Autodesk Inventor part; units mm, degrees
(part 2 of 3)
  line L279 (-5.846, -1.6903) -> (-6.0548, -1.6903)
  line L280 (-6.0548, -1.6903) -> (-6.3396, -0.5285)
  line L281 (-6.3396, -0.5285) -> (-6.6164, -1.6903)
  line L282 (-6.6164, -1.6903) -> (-6.8229, -1.6903)
  line L283 (-6.8229, -1.6903) -> (-7.1802, -0.2903)
  line L284 (-7.1802, -0.2903) -> (-6.9885, -0.2903)
  line L285 (-6.9885, -0.2903) -> (-6.7071, -1.4509)
  line L286 (-6.7071, -1.4509) -> (-6.4281, -0.2903)
  line L287 (-6.4281, -0.2903) -> (-6.2386, -0.2903)
  line L288 (-6.2386, -0.2903) -> (-5.9572, -1.4645)
  line L289 (-5.9572, -1.4645) -> (-5.677, -0.2903)
  line L290 (-5.677, -0.2903) -> (-5.4943, -0.2903)
  spline S281 degree 2 poles (-4.7558, -1.5791) (-4.7773, -1.595) (-4.8499, -1.6517) (-4.884, -1.6687) knots 0 0 0 1 2 2 2
  spline S282 degree 2 poles (-4.884, -1.6687) (-4.9305, -1.6937) (-5.0178, -1.7198) (-5.0973, -1.7198) knots 0 0 0 1 2 2 2
  spline S283 degree 2 poles (-5.0973, -1.7198) (-5.1619, -1.7198) (-5.2788, -1.671) (-5.323, -1.6268) knots 0 0 0 1 2 2 2
  spline S284 degree 2 poles (-5.323, -1.6268) (-5.365, -1.5836) (-5.4161, -1.4566) (-5.4161, -1.3862) knots 0 0 0 1 2 2 2
  spline S285 degree 2 poles (-5.4161, -1.3862) (-5.4161, -1.2773) (-5.3242, -1.123) (-5.2243, -1.0788) knots 0 0 0 1 2 2 2
  spline S286 degree 2 poles (-5.2243, -1.0788) (-5.1358, -1.0379) (-4.8953, -1.0073) (-4.7558, -0.9994) knots 0 0 0 1 2 2 2
  line L291 (-4.7558, -0.9994) -> (-4.7558, -0.9653)
  spline S287 degree 2 poles (-4.7558, -0.9653) (-4.7558, -0.9041) (-4.7932, -0.8281) (-4.8272, -0.8065) knots 0 0 0 1 2 2 2
  spline S288 degree 2 poles (-4.8272, -0.8065) (-4.8613, -0.7849) (-4.9588, -0.7713) (-5.011, -0.7713) knots 0 0 0 1 2 2 2
  spline S289 degree 2 poles (-5.011, -0.7713) (-5.0723, -0.7713) (-5.2379, -0.8076) (-5.3208, -0.8428) knots 0 0 0 1 2 2 2
  line L292 (-5.3208, -0.8428) -> (-5.331, -0.8428)
  line L293 (-5.331, -0.8428) -> (-5.331, -0.6624)
  spline S290 degree 2 poles (-5.331, -0.6624) (-5.2822, -0.6488) (-5.0995, -0.6148) (-5.0099, -0.6148) knots 0 0 0 1 2 2 2
  spline S291 degree 2 poles (-5.0099, -0.6148) (-4.901, -0.6148) (-4.7524, -0.6488) (-4.6934, -0.6931) knots 0 0 0 1 2 2 2
  spline S292 degree 2 poles (-4.6934, -0.6931) (-4.6355, -0.7362) (-4.5788, -0.8734) (-4.5788, -0.9721) knots 0 0 0 1 2 2 2
  line L294 (-4.5788, -0.9721) -> (-4.5788, -1.6903)
  line L295 (-4.5788, -1.6903) -> (-4.7558, -1.6903)
  line L296 (-4.7558, -1.6903) -> (-4.7558, -1.5791)
  line L297 (-4.7558, -1.4316) -> (-4.7558, -1.1401)
  spline S293 degree 2 poles (-4.7558, -1.1401) (-4.8193, -1.1457) (-5.011, -1.165) (-5.0712, -1.1832) knots 0 0 0 1 2 2 2
  spline S294 degree 2 poles (-5.0712, -1.1832) (-5.1415, -1.2047) (-5.2334, -1.2943) (-5.2334, -1.3738) knots 0 0 0 1 2 2 2
  spline S295 degree 2 poles (-5.2334, -1.3738) (-5.2334, -1.4645) (-5.1313, -1.5564) (-5.0337, -1.5564) knots 0 0 0 1 2 2 2
  spline S296 degree 2 poles (-5.0337, -1.5564) (-4.9509, -1.5564) (-4.8148, -1.4849) (-4.7558, -1.4316) knots 0 0 0 1 2 2 2
  line L298 (-3.5055, -0.6397) -> (-3.9015, -1.6903)
  line L299 (-3.9015, -1.6903) -> (-4.0603, -1.6903)
  line L300 (-4.0603, -1.6903) -> (-4.4529, -0.6397)
  line L301 (-4.4529, -0.6397) -> (-4.2611, -0.6397)
  line L302 (-4.2611, -0.6397) -> (-3.9741, -1.4486)
  line L303 (-3.9741, -1.4486) -> (-3.6893, -0.6397)
  line L304 (-3.6893, -0.6397) -> (-3.5055, -0.6397)
  spline S297 degree 2 poles (-2.9156, -1.7141) (-3.1674, -1.7141) (-3.4443, -1.4316) (-3.4443, -1.1707) knots 0 0 0 1 2 2 2
  spline S298 degree 2 poles (-3.4443, -1.1707) (-3.4443, -0.9143) (-3.1754, -0.6102) (-2.9587, -0.6102) knots 0 0 0 1 2 2 2
  spline S299 degree 2 poles (-2.9587, -0.6102) (-2.8611, -0.6102) (-2.7102, -0.667) (-2.6546, -0.7271) knots 0 0 0 1 2 2 2
  spline S300 degree 2 poles (-2.6546, -0.7271) (-2.5979, -0.7872) (-2.5378, -0.9608) (-2.5378, -1.0867) knots 0 0 0 1 2 2 2
  line L305 (-2.5378, -1.0867) -> (-2.5378, -1.1832)
  line L306 (-2.5378, -1.1832) -> (-3.265, -1.1832)
  spline S301 degree 2 poles (-3.265, -1.1832) (-3.265, -1.3658) (-3.0812, -1.5598) (-2.9178, -1.5598) knots 0 0 0 1 2 2 2
  spline S302 degree 2 poles (-2.9178, -1.5598) (-2.86, -1.5598) (-2.7477, -1.5337) (-2.7023, -1.5133) knots 0 0 0 1 2 2 2
  spline S303 degree 2 poles (-2.7023, -1.5133) (-2.6546, -1.4906) (-2.5888, -1.4509) (-2.5673, -1.4328) knots 0 0 0 1 2 2 2
  line L307 (-2.5673, -1.4328) -> (-2.5571, -1.4328)
  line L308 (-2.5571, -1.4328) -> (-2.5571, -1.6256)
  spline S304 degree 2 poles (-2.5571, -1.6256) (-2.5877, -1.6381) (-2.6807, -1.6744) (-2.717, -1.6846) knots 0 0 0 1 2 2 2
  spline S305 degree 2 poles (-2.717, -1.6846) (-2.7681, -1.6994) (-2.852, -1.7141) (-2.9156, -1.7141) knots 0 0 0 1 2 2 2
  spline S306 degree 2 poles (-2.7102, -1.0482) (-2.7125, -0.9767) (-2.742, -0.8723) (-2.7704, -0.8371) knots 0 0 0 1 2 2 2
  spline S307 degree 2 poles (-2.7704, -0.8371) (-2.801, -0.7974) (-2.8974, -0.7554) (-2.9689, -0.7554) knots 0 0 0 1 2 2 2
  spline S308 degree 2 poles (-2.9689, -0.7554) (-3.0392, -0.7554) (-3.1379, -0.7974) (-3.1788, -0.8383) knots 0 0 0 1 2 2 2
  spline S309 degree 2 poles (-3.1788, -0.8383) (-3.2185, -0.8802) (-3.2593, -0.9812) (-3.265, -1.0482) knots 0 0 0 1 2 2 2
  line L309 (-3.265, -1.0482) -> (-2.7102, -1.0482)
  line L310 (-2.1781, -1.6903) -> (-2.3551, -1.6903)
  line L311 (-2.3551, -1.6903) -> (-2.3551, -0.2279)
  line L312 (-2.3551, -0.2279) -> (-2.1781, -0.2279)
  line L313 (-2.1781, -0.2279) -> (-2.1781, -1.6903)
  spline S310 degree 2 poles (-1.4623, -1.7141) (-1.7141, -1.7141) (-1.9909, -1.4316) (-1.9909, -1.1707) knots 0 0 0 1 2 2 2
  spline S311 degree 2 poles (-1.9909, -1.1707) (-1.9909, -0.9143) (-1.7221, -0.6102) (-1.5054, -0.6102) knots 0 0 0 1 2 2 2
  spline S312 degree 2 poles (-1.5054, -0.6102) (-1.4078, -0.6102) (-1.2569, -0.667) (-1.2013, -0.7271) knots 0 0 0 1 2 2 2
  spline S313 degree 2 poles (-1.2013, -0.7271) (-1.1446, -0.7872) (-1.0845, -0.9608) (-1.0845, -1.0867) knots 0 0 0 1 2 2 2
  line L314 (-1.0845, -1.0867) -> (-1.0845, -1.1832)
  line L315 (-1.0845, -1.1832) -> (-1.8117, -1.1832)
  spline S314 degree 2 poles (-1.8117, -1.1832) (-1.8117, -1.3658) (-1.6279, -1.5598) (-1.4645, -1.5598) knots 0 0 0 1 2 2 2
  spline S315 degree 2 poles (-1.4645, -1.5598) (-1.4067, -1.5598) (-1.2943, -1.5337) (-1.249, -1.5133) knots 0 0 0 1 2 2 2
  spline S316 degree 2 poles (-1.249, -1.5133) (-1.2013, -1.4906) (-1.1355, -1.4509) (-1.114, -1.4328) knots 0 0 0 1 2 2 2
  line L316 (-1.114, -1.4328) -> (-1.1037, -1.4328)
  line L317 (-1.1037, -1.4328) -> (-1.1037, -1.6256)
  spline S317 degree 2 poles (-1.1037, -1.6256) (-1.1344, -1.6381) (-1.2274, -1.6744) (-1.2637, -1.6846) knots 0 0 0 1 2 2 2
  spline S318 degree 2 poles (-1.2637, -1.6846) (-1.3148, -1.6994) (-1.3987, -1.7141) (-1.4623, -1.7141) knots 0 0 0 1 2 2 2
  spline S319 degree 2 poles (-1.2569, -1.0482) (-1.2592, -0.9767) (-1.2887, -0.8723) (-1.317, -0.8371) knots 0 0 0 1 2 2 2
  spline S320 degree 2 poles (-1.317, -0.8371) (-1.3477, -0.7974) (-1.4441, -0.7554) (-1.5156, -0.7554) knots 0 0 0 1 2 2 2
  spline S321 degree 2 poles (-1.5156, -0.7554) (-1.5859, -0.7554) (-1.6846, -0.7974) (-1.7255, -0.8383) knots 0 0 0 1 2 2 2
  spline S322 degree 2 poles (-1.7255, -0.8383) (-1.7652, -0.8802) (-1.806, -0.9812) (-1.8117, -1.0482) knots 0 0 0 1 2 2 2
  line L318 (-1.8117, -1.0482) -> (-1.2569, -1.0482)
  line L319 (-0.0804, -1.6903) -> (-0.2574, -1.6903)
  line L320 (-0.2574, -1.6903) -> (-0.2574, -1.0913)
  spline S323 degree 2 poles (-0.2574, -1.0913) (-0.2574, -1.0187) (-0.271, -0.8939) (-0.2914, -0.8564) knots 0 0 0 1 2 2 2
  spline S324 degree 2 poles (-0.2914, -0.8564) (-0.313, -0.8167) (-0.3901, -0.7781) (-0.4559, -0.7781) knots 0 0 0 1 2 2 2
  spline S325 degree 2 poles (-0.4559, -0.7781) (-0.5217, -0.7781) (-0.6613, -0.8485) (-0.7282, -0.9052) knots 0 0 0 1 2 2 2
  line L321 (-0.7282, -0.9052) -> (-0.7282, -1.6903)
  line L322 (-0.7282, -1.6903) -> (-0.9052, -1.6903)
  line L323 (-0.9052, -1.6903) -> (-0.9052, -0.6397)
  line L324 (-0.9052, -0.6397) -> (-0.7282, -0.6397)
  line L325 (-0.7282, -0.6397) -> (-0.7282, -0.7566)
  spline S326 degree 2 poles (-0.7282, -0.7566) (-0.6488, -0.6851) (-0.4956, -0.6102) (-0.4094, -0.6102) knots 0 0 0 1 2 2 2
  spline S327 degree 2 poles (-0.4094, -0.6102) (-0.2551, -0.6102) (-0.0804, -0.8144) (-0.0804, -1.0084) knots 0 0 0 1 2 2 2
  line L326 (-0.0804, -1.0084) -> (-0.0804, -1.6903)
  spline S328 degree 2 poles (0.2055, -1.8582) (0.2236, -1.8661) (0.2929, -1.8911) (0.3371, -1.9013) knots 0 0 0 1 2 2 2
  spline S329 degree 2 poles (0.3371, -1.9013) (0.3859, -1.9138) (0.4687, -1.9285) (0.5175, -1.9285) knots 0 0 0 1 2 2 2
  spline S330 degree 2 poles (0.5175, -1.9285) (0.5992, -1.9285) (0.7126, -1.8854) (0.7444, -1.8469) knots 0 0 0 1 2 2 2
  spline S331 degree 2 poles (0.7444, -1.8469) (0.775, -1.8083) (0.7989, -1.7073) (0.7989, -1.6426) knots 0 0 0 1 2 2 2
  line L327 (0.7989, -1.6426) -> (0.7989, -1.5507)
  spline S332 degree 2 poles (0.7989, -1.5507) (0.7274, -1.6131) (0.5901, -1.6721) (0.4869, -1.6721) knots 0 0 0 1 2 2 2
  spline S333 degree 2 poles (0.4869, -1.6721) (0.3076, -1.6721) (0.0954, -1.4055) (0.0954, -1.1548) knots 0 0 0 1 2 2 2
  spline S334 degree 2 poles (0.0954, -1.1548) (0.0954, -1.0243) (0.1692, -0.8224) (0.2305, -0.7509) knots 0 0 0 1 2 2 2
  spline S335 degree 2 poles (0.2305, -0.7509) (0.2895, -0.684) (0.4517, -0.6102) (0.5379, -0.6102) knots 0 0 0 1 2 2 2
  spline S336 degree 2 poles (0.5379, -0.6102) (0.6196, -0.6102) (0.7387, -0.6488) (0.7989, -0.684) knots 0 0 0 1 2 2 2
  line L328 (0.7989, -0.684) -> (0.8091, -0.6397)
  line L329 (0.8091, -0.6397) -> (0.9758, -0.6397)
  line L330 (0.9758, -0.6397) -> (0.9758, -1.57)
  spline S337 degree 2 poles (0.9758, -1.57) (0.9758, -1.8378) (0.7433, -2.0874) (0.5039, -2.0874) knots 0 0 0 1 2 2 2
  spline S338 degree 2 poles (0.5039, -2.0874) (0.4267, -2.0874) (0.2656, -2.0624) (0.1964, -2.042) knots 0 0 0 1 2 2 2
  line L331 (0.1964, -2.042) -> (0.1964, -1.8582)
  line L332 (0.1964, -1.8582) -> (0.2055, -1.8582)
  line L333 (0.7989, -1.4055) -> (0.7989, -0.8281)
  spline S339 degree 2 poles (0.7989, -0.8281) (0.733, -0.7963) (0.6219, -0.7691) (0.5663, -0.7691) knots 0 0 0 1 2 2 2
  spline S340 degree 2 poles (0.5663, -0.7691) (0.4324, -0.7691) (0.2781, -0.9665) (0.2781, -1.1514) knots 0 0 0 1 2 2 2
  spline S341 degree 2 poles (0.2781, -1.1514) (0.2781, -1.3261) (0.395, -1.5088) (0.5266, -1.5088) knots 0 0 0 1 2 2 2
  spline S342 degree 2 poles (0.5266, -1.5088) (0.5958, -1.5088) (0.741, -1.4543) (0.7989, -1.4055) knots 0 0 0 1 2 2 2
  spline S343 degree 2 poles (1.5499, -1.7107) (1.4058, -1.7107) (1.2436, -1.5462) (1.2436, -1.3681) knots 0 0 0 1 2 2 2
  line L334 (1.2436, -1.3681) -> (1.2436, -0.7861)
  line L335 (1.2436, -0.7861) -> (1.1245, -0.7861)
  line L336 (1.1245, -0.7861) -> (1.1245, -0.6397)
  line L337 (1.1245, -0.6397) -> (1.2436, -0.6397)
  line L338 (1.2436, -0.6397) -> (1.2436, -0.3379)
  line L339 (1.2436, -0.3379) -> (1.4206, -0.3379)
  line L340 (1.4206, -0.3379) -> (1.4206, -0.6397)
  line L341 (1.4206, -0.6397) -> (1.7462, -0.6397)
  line L342 (1.7462, -0.6397) -> (1.7462, -0.7861)
  line L343 (1.7462, -0.7861) -> (1.4206, -0.7861)
  line L344 (1.4206, -0.7861) -> (1.4206, -1.2864)
  spline S344 degree 2 poles (1.4206, -1.2864) (1.4206, -1.3658) (1.4262, -1.4532) (1.4455, -1.4906) knots 0 0 0 1 2 2 2
  spline S345 degree 2 poles (1.4455, -1.4906) (1.4614, -1.5235) (1.5329, -1.5564) (1.5942, -1.5564) knots 0 0 0 1 2 2 2
  spline S346 degree 2 poles (1.5942, -1.5564) (1.6373, -1.5564) (1.7178, -1.5303) (1.736, -1.5224) knots 0 0 0 1 2 2 2
  line L345 (1.736, -1.5224) -> (1.7462, -1.5224)
  line L346 (1.7462, -1.5224) -> (1.7462, -1.6812)
  spline S347 degree 2 poles (1.7462, -1.6812) (1.6963, -1.6948) (1.5942, -1.7107) (1.5499, -1.7107) knots 0 0 0 1 2 2 2
  line L347 (2.7014, -1.6903) -> (2.5245, -1.6903)
  line L348 (2.5245, -1.6903) -> (2.5245, -1.0913)
  spline S348 degree 2 poles (2.5245, -1.0913) (2.5245, -1.0187) (2.5108, -0.8939) (2.4904, -0.8564) knots 0 0 0 1 2 2 2
  spline S349 degree 2 poles (2.4904, -0.8564) (2.4689, -0.8167) (2.3917, -0.7781) (2.3259, -0.7781) knots 0 0 0 1 2 2 2
  spline S350 degree 2 poles (2.3259, -0.7781) (2.2601, -0.7781) (2.1206, -0.8485) (2.0536, -0.9052) knots 0 0 0 1 2 2 2
  line L349 (2.0536, -0.9052) -> (2.0536, -1.6903)
  line L350 (2.0536, -1.6903) -> (1.8766, -1.6903)
  line L351 (1.8766, -1.6903) -> (1.8766, -0.2279)
  line L352 (1.8766, -0.2279) -> (2.0536, -0.2279)
  line L353 (2.0536, -0.2279) -> (2.0536, -0.7566)
  spline S351 degree 2 poles (2.0536, -0.7566) (2.133, -0.6851) (2.2862, -0.6102) (2.3724, -0.6102) knots 0 0 0 1 2 2 2
  spline S352 degree 2 poles (2.3724, -0.6102) (2.5267, -0.6102) (2.7014, -0.8144) (2.7014, -1.0084) knots 0 0 0 1 2 2 2
  line L354 (2.7014, -1.0084) -> (2.7014, -1.6903)
  line L355 (3.8757, -1.6903) -> (3.651, -1.6903)
  line L356 (3.651, -1.6903) -> (3.651, -1.4225)
  line L357 (3.651, -1.4225) -> (3.8757, -1.4225)
  line L358 (3.8757, -1.4225) -> (3.8757, -1.6903)
  line L359 (3.8757, -0.9075) -> (3.651, -0.9075)
  line L360 (3.651, -0.9075) -> (3.651, -0.6397)
  line L361 (3.651, -0.6397) -> (3.8757, -0.6397)
  line L362 (3.8757, -0.6397) -> (3.8757, -0.9075)
  spline S353 degree 2 poles (5.692, -1.2365) (5.692, -1.3443) (5.6206, -1.5269) (5.5604, -1.5882) knots 0 0 0 1 2 2 2
  spline S354 degree 2 poles (5.5604, -1.5882) (5.498, -1.6529) (5.3415, -1.7198) (5.2473, -1.7198) knots 0 0 0 1 2 2 2
  spline S355 degree 2 poles (5.2473, -1.7198) (5.1531, -1.7198) (4.9977, -1.6563) (4.9387, -1.5927) knots 0 0 0 1 2 2 2
  spline S356 degree 2 poles (4.9387, -1.5927) (4.8661, -1.5167) (4.7844, -1.2614) (4.7844, -1.0754) knots 0 0 0 1 2 2 2
  spline S357 degree 2 poles (4.7844, -1.0754) (4.7844, -0.8927) (4.8593, -0.5989) (4.9376, -0.49) knots 0 0 0 1 2 2 2
  spline S358 degree 2 poles (4.9376, -0.49) (5.0136, -0.3833) (5.2541, -0.2642) (5.4118, -0.2642) knots 0 0 0 1 2 2 2
  spline S359 degree 2 poles (5.4118, -0.2642) (5.4583, -0.2642) (5.54, -0.2733) (5.5707, -0.2835) knots 0 0 0 1 2 2 2
  line L363 (5.5707, -0.2835) -> (5.5707, -0.4639)
  line L364 (5.5707, -0.4639) -> (5.5627, -0.4639)
  spline S360 degree 2 poles (5.5627, -0.4639) (5.5366, -0.4503) (5.4413, -0.4264) (5.3869, -0.4264) knots 0 0 0 1 2 2 2
  spline S361 degree 2 poles (5.3869, -0.4264) (5.2121, -0.4264) (4.9977, -0.6624) (4.9773, -0.8939) knots 0 0 0 1 2 2 2
  spline S362 degree 2 poles (4.9773, -0.8939) (5.0442, -0.8473) (5.1849, -0.7963) (5.2689, -0.7963) knots 0 0 0 1 2 2 2
  spline S363 degree 2 poles (5.2689, -0.7963) (5.3506, -0.7963) (5.4731, -0.8292) (5.54, -0.8791) knots 0 0 0 1 2 2 2
  spline S364 degree 2 poles (5.54, -0.8791) (5.6172, -0.937) (5.692, -1.1162) (5.692, -1.2365) knots 0 0 0 1 2 2 2
  spline S365 degree 2 poles (5.5014, -1.2444) (5.5014, -1.1582) (5.4561, -1.0413) (5.4061, -1.0005) knots 0 0 0 1 2 2 2
  spline S366 degree 2 poles (5.4061, -1.0005) (5.3687, -0.971) (5.2757, -0.9517) (5.2269, -0.9517) knots 0 0 0 1 2 2 2
  spline S367 degree 2 poles (5.2269, -0.9517) (5.1611, -0.9517) (5.0374, -0.9914) (4.9773, -1.0289) knots 0 0 0 1 2 2 2
  spline S368 degree 2 poles (4.9773, -1.0289) (4.9762, -1.0493) (4.9739, -1.0879) (4.9739, -1.1174) knots 0 0 0 1 2 2 2
  spline S369 degree 2 poles (4.9739, -1.1174) (4.9739, -1.2626) (5.0306, -1.4407) (5.0737, -1.4872) knots 0 0 0 1 2 2 2
  spline S370 degree 2 poles (5.0737, -1.4872) (5.1134, -1.5315) (5.1997, -1.5666) (5.2484, -1.5666) knots 0 0 0 1 2 2 2
  spline S371 degree 2 poles (5.2484, -1.5666) (5.3619, -1.5666) (5.5014, -1.4055) (5.5014, -1.2444) knots 0 0 0 1 2 2 2
  spline S372 degree 2 poles (6.2355, -0.423) (6.1844, -0.423) (6.0835, -0.448) (6.0347, -0.4673) knots 0 0 0 1 2 2 2
  spline S373 degree 2 poles (6.0347, -0.4673) (5.9893, -0.4866) (5.9224, -0.5274) (5.8963, -0.5456) knots 0 0 0 1 2 2 2
  line L365 (5.8963, -0.5456) -> (5.8849, -0.5456)
  line L366 (5.8849, -0.5456) -> (5.8849, -0.347)
  spline S374 degree 2 poles (5.8849, -0.347) (5.9462, -0.3141) (6.1561, -0.2608) (6.2502, -0.2608) knots 0 0 0 1 2 2 2
  spline S375 degree 2 poles (6.2502, -0.2608) (6.3455, -0.2608) (6.4873, -0.2994) (6.5452, -0.3402) knots 0 0 0 1 2 2 2
  spline S376 degree 2 poles (6.5452, -0.3402) (6.6065, -0.3845) (6.67, -0.5127) (6.67, -0.5989) knots 0 0 0 1 2 2 2
  spline S377 degree 2 poles (6.67, -0.5989) (6.67, -0.7146) (6.518, -0.8893) (6.4113, -0.912) knots 0 0 0 1 2 2 2
  line L367 (6.4113, -0.912) -> (6.4113, -0.9256)
  spline S378 degree 2 poles (6.4113, -0.9256) (6.4556, -0.9347) (6.5565, -0.9755) (6.5997, -1.0164) knots 0 0 0 1 2 2 2
  spline S379 degree 2 poles (6.5997, -1.0164) (6.6428, -1.0561) (6.6972, -1.1832) (6.6972, -1.2751) knots 0 0 0 1 2 2 2
  spline S380 degree 2 poles (6.6972, -1.2751) (6.6972, -1.3692) (6.6326, -1.5292) (6.5736, -1.5905) knots 0 0 0 1 2 2 2
  spline S381 degree 2 poles (6.5736, -1.5905) (6.5123, -1.654) (6.3387, -1.7198) (6.2287, -1.7198) knots 0 0 0 1 2 2 2
  spline S382 degree 2 poles (6.2287, -1.7198) (6.1232, -1.7198) (5.9167, -1.6687) (5.8463, -1.6336) knots 0 0 0 1 2 2 2
  line L368 (5.8463, -1.6336) -> (5.8463, -1.435)
  line L369 (5.8463, -1.435) -> (5.86, -1.435)
  spline S383 degree 2 poles (5.86, -1.435) (5.9189, -1.4781) (6.1186, -1.5576) (6.2173, -1.5576) knots 0 0 0 1 2 2 2
  spline S384 degree 2 poles (6.2173, -1.5576) (6.2752, -1.5576) (6.3909, -1.5213) (6.4295, -1.4793) knots 0 0 0 1 2 2 2
  spline S385 degree 2 poles (6.4295, -1.4793) (6.4669, -1.4373) (6.5066, -1.3375) (6.5066, -1.2614) knots 0 0 0 1 2 2 2
  spline S386 degree 2 poles (6.5066, -1.2614) (6.5066, -1.1854) (6.4624, -1.0867) (6.4227, -1.0584) knots 0 0 0 1 2 2 2
  spline S387 degree 2 poles (6.4227, -1.0584) (6.383, -1.03) (6.2752, -1.0084) (6.2117, -1.0084) knots 0 0 0 1 2 2 2
  line L370 (6.2117, -1.0084) -> (6.1322, -1.0084)
  line L371 (6.1322, -1.0084) -> (6.1322, -0.853)
  line L372 (6.1322, -0.853) -> (6.1946, -0.853)
  spline S388 degree 2 poles (6.1946, -0.853) (6.3206, -0.853) (6.4794, -0.7328) (6.4794, -0.6182) knots 0 0 0 1 2 2 2
  spline S389 degree 2 poles (6.4794, -0.6182) (6.4794, -0.5648) (6.4386, -0.4888) (6.4057, -0.4661) knots 0 0 0 1 2 2 2
  spline S390 degree 2 poles (6.4057, -0.4661) (6.3705, -0.4423) (6.2843, -0.423) (6.2355, -0.423) knots 0 0 0 1 2 2 2
  spline S391 degree 2 poles (7.7932, -1.2365) (7.7932, -1.3443) (7.7217, -1.5269) (7.6616, -1.5882) knots 0 0 0 1 2 2 2
  spline S392 degree 2 poles (7.6616, -1.5882) (7.5992, -1.6529) (7.4426, -1.7198) (7.3484, -1.7198) knots 0 0 0 1 2 2 2
  spline S393 degree 2 poles (7.3484, -1.7198) (7.2543, -1.7198) (7.0989, -1.6563) (7.0399, -1.5927) knots 0 0 0 1 2 2 2
  spline S394 degree 2 poles (7.0399, -1.5927) (6.9672, -1.5167) (6.8856, -1.2614) (6.8856, -1.0754) knots 0 0 0 1 2 2 2
  spline S395 degree 2 poles (6.8856, -1.0754) (6.8856, -0.8927) (6.9604, -0.5989) (7.0387, -0.49) knots 0 0 0 1 2 2 2
  spline S396 degree 2 poles (7.0387, -0.49) (7.1147, -0.3833) (7.3553, -0.2642) (7.513, -0.2642) knots 0 0 0 1 2 2 2
  spline S397 degree 2 poles (7.513, -0.2642) (7.5595, -0.2642) (7.6412, -0.2733) (7.6718, -0.2835) knots 0 0 0 1 2 2 2
  line L373 (7.6718, -0.2835) -> (7.6718, -0.4639)
  line L374 (7.6718, -0.4639) -> (7.6638, -0.4639)
  spline S398 degree 2 poles (7.6638, -0.4639) (7.6377, -0.4503) (7.5424, -0.4264) (7.488, -0.4264) knots 0 0 0 1 2 2 2
  spline S399 degree 2 poles (7.488, -0.4264) (7.3133, -0.4264) (7.0989, -0.6624) (7.0784, -0.8939) knots 0 0 0 1 2 2 2
  spline S400 degree 2 poles (7.0784, -0.8939) (7.1454, -0.8473) (7.286, -0.7963) (7.37, -0.7963) knots 0 0 0 1 2 2 2
  spline S401 degree 2 poles (7.37, -0.7963) (7.4517, -0.7963) (7.5742, -0.8292) (7.6412, -0.8791) knots 0 0 0 1 2 2 2
  spline S402 degree 2 poles (7.6412, -0.8791) (7.7183, -0.937) (7.7932, -1.1162) (7.7932, -1.2365) knots 0 0 0 1 2 2 2
  spline S403 degree 2 poles (7.6026, -1.2444) (7.6026, -1.1582) (7.5572, -1.0413) (7.5073, -1.0005) knots 0 0 0 1 2 2 2
  spline S404 degree 2 poles (7.5073, -1.0005) (7.4698, -0.971) (7.3768, -0.9517) (7.328, -0.9517) knots 0 0 0 1 2 2 2
  spline S405 degree 2 poles (7.328, -0.9517) (7.2622, -0.9517) (7.1386, -0.9914) (7.0784, -1.0289) knots 0 0 0 1 2 2 2
  spline S406 degree 2 poles (7.0784, -1.0289) (7.0773, -1.0493) (7.075, -1.0879) (7.075, -1.1174) knots 0 0 0 1 2 2 2
  spline S407 degree 2 poles (7.075, -1.1174) (7.075, -1.2626) (7.1318, -1.4407) (7.1749, -1.4872) knots 0 0 0 1 2 2 2
  spline S408 degree 2 poles (7.1749, -1.4872) (7.2146, -1.5315) (7.3008, -1.5666) (7.3496, -1.5666) knots 0 0 0 1 2 2 2
  spline S409 degree 2 poles (7.3496, -1.5666) (7.463, -1.5666) (7.6026, -1.4055) (7.6026, -1.2444) knots 0 0 0 1 2 2 2
  line L375 (8.2595, -1.6903) -> (8.0348, -1.6903)
  line L376 (8.0348, -1.6903) -> (8.0348, -1.4225)
  line L377 (8.0348, -1.4225) -> (8.2595, -1.4225)
  line L378 (8.2595, -1.4225) -> (8.2595, -1.6903)
  spline S410 degree 2 poles (8.5034, -0.7452) (8.5034, -0.6375) (8.5737, -0.4582) (8.635, -0.3935) knots 0 0 0 1 2 2 2
  spline S411 degree 2 poles (8.635, -0.3935) (8.6929, -0.3311) (8.8619, -0.2619) (8.9481, -0.2619) knots 0 0 0 1 2 2 2
  spline S412 degree 2 poles (8.9481, -0.2619) (9.0446, -0.2619) (9.2011, -0.3266) (9.259, -0.3879) knots 0 0 0 1 2 2 2
  spline S413 degree 2 poles (9.259, -0.3879) (9.3316, -0.465) (9.411, -0.7146) (9.411, -0.9063) knots 0 0 0 1 2 2 2
  spline S414 degree 2 poles (9.411, -0.9063) (9.411, -1.0799) (9.3327, -1.3908) (9.2567, -1.494) knots 0 0 0 1 2 2 2
  spline S415 degree 2 poles (9.2567, -1.494) (9.1762, -1.6029) (8.9493, -1.7175) (8.7836, -1.7175) knots 0 0 0 1 2 2 2
  spline S416 degree 2 poles (8.7836, -1.7175) (8.7462, -1.7175) (8.6611, -1.7096) (8.6248, -1.6982) knots 0 0 0 1 2 2 2
  line L379 (8.6248, -1.6982) -> (8.6248, -1.5178)
  line L380 (8.6248, -1.5178) -> (8.6339, -1.5178)
  spline S417 degree 2 poles (8.6339, -1.5178) (8.6577, -1.5315) (8.7575, -1.5553) (8.8086, -1.5553) knots 0 0 0 1 2 2 2
  spline S418 degree 2 poles (8.8086, -1.5553) (8.9924, -1.5553) (9.2023, -1.3125) (9.217, -1.0879) knots 0 0 0 1 2 2 2
  spline S419 degree 2 poles (9.217, -1.0879) (9.1421, -1.1389) (9.006, -1.1854) (8.9254, -1.1854) knots 0 0 0 1 2 2 2
  spline S420 degree 2 poles (8.9254, -1.1854) (8.8483, -1.1854) (8.7201, -1.1514) (8.6554, -1.1026) knots 0 0 0 1 2 2 2
  spline S421 degree 2 poles (8.6554, -1.1026) (8.5805, -1.0448) (8.5034, -0.8689) (8.5034, -0.7452) knots 0 0 0 1 2 2 2
  spline S422 degree 2 poles (9.2215, -0.8644) (9.2215, -0.7225) (9.1694, -0.5433) (9.1228, -0.4945) knots 0 0 0 1 2 2 2
  spline S423 degree 2 poles (9.1228, -0.4945) (9.082, -0.4491) (8.9969, -0.4151) (8.947, -0.4151) knots 0 0 0 1 2 2 2
  spline S424 degree 2 poles (8.947, -0.4151) (8.8313, -0.4151) (8.694, -0.5807) (8.694, -0.7373) knots 0 0 0 1 2 2 2
  spline S425 degree 2 poles (8.694, -0.7373) (8.694, -0.8258) (8.7394, -0.9404) (8.7893, -0.9812) knots 0 0 0 1 2 2 2
  spline S426 degree 2 poles (8.7893, -0.9812) (8.8256, -1.0107) (8.9152, -1.03) (8.9674, -1.03) knots 0 0 0 1 2 2 2
  spline S427 degree 2 poles (8.9674, -1.03) (9.0275, -1.03) (9.166, -0.988) (9.2181, -0.9529) knots 0 0 0 1 2 2 2
  spline S428 degree 2 poles (9.2181, -0.9529) (9.2193, -0.9392) (9.2215, -0.8927) (9.2215, -0.8644) knots 0 0 0 1 2 2 2
  line L381 (11.0447, -1.6903) -> (10.8677, -1.6903)
  line L382 (10.8677, -1.6903) -> (10.8677, -1.0913)
  spline S429 degree 2 poles (10.8677, -1.0913) (10.8677, -1.0187) (10.8541, -0.8939) (10.8337, -0.8564) knots 0 0 0 1 2 2 2
  spline S430 degree 2 poles (10.8337, -0.8564) (10.8121, -0.8167) (10.735, -0.7781) (10.6692, -0.7781) knots 0 0 0 1 2 2 2
  spline S431 degree 2 poles (10.6692, -0.7781) (10.6034, -0.7781) (10.4638, -0.8485) (10.3969, -0.9052) knots 0 0 0 1 2 2 2
  line L383 (10.3969, -0.9052) -> (10.3969, -1.6903)
  line L384 (10.3969, -1.6903) -> (10.2199, -1.6903)
  line L385 (10.2199, -1.6903) -> (10.2199, -0.6397)
  line L386 (10.2199, -0.6397) -> (10.3969, -0.6397)
  line L387 (10.3969, -0.6397) -> (10.3969, -0.7566)
  spline S432 degree 2 poles (10.3969, -0.7566) (10.4763, -0.6851) (10.6295, -0.6102) (10.7157, -0.6102) knots 0 0 0 1 2 2 2
  spline S433 degree 2 poles (10.7157, -0.6102) (10.87, -0.6102) (11.0447, -0.8144) (11.0447, -1.0084) knots 0 0 0 1 2 2 2
  line L388 (11.0447, -1.0084) -> (11.0447, -1.6903)
  line L389 (12.4844, -1.6903) -> (12.4844, -1.0822)
  spline S434 degree 2 poles (12.4844, -1.0822) (12.4844, -1.0096) (12.4731, -0.8859) (12.4549, -0.8519) knots 0 0 0 1 2 2 2
  spline S435 degree 2 poles (12.4549, -0.8519) (12.4368, -0.8144) (12.3676, -0.7781) (12.3074, -0.7781) knots 0 0 0 1 2 2 2
  spline S436 degree 2 poles (12.3074, -0.7781) (12.253, -0.7781) (12.1282, -0.8451) (12.0624, -0.9086) knots 0 0 0 1 2 2 2
  spline S437 degree 2 poles (12.0624, -0.9086) (12.0635, -0.9245) (12.0658, -0.9687) (12.0658, -0.9982) knots 0 0 0 1 2 2 2
  line L390 (12.0658, -0.9982) -> (12.0658, -1.6903)
  line L391 (12.0658, -1.6903) -> (11.8888, -1.6903)
  line L392 (11.8888, -1.6903) -> (11.8888, -1.0822)
  spline S438 degree 2 poles (11.8888, -1.0822) (11.8888, -1.0096) (11.8775, -0.8859) (11.8593, -0.8519) knots 0 0 0 1 2 2 2
  spline S439 degree 2 poles (11.8593, -0.8519) (11.8412, -0.8144) (11.7719, -0.7781) (11.7118, -0.7781) knots 0 0 0 1 2 2 2
  spline S440 degree 2 poles (11.7118, -0.7781) (11.6551, -0.7781) (11.5292, -0.8496) (11.4702, -0.9052) knots 0 0 0 1 2 2 2
  line L393 (11.4702, -0.9052) -> (11.4702, -1.6903)
  line L394 (11.4702, -1.6903) -> (11.2932, -1.6903)
  line L395 (11.2932, -1.6903) -> (11.2932, -0.6397)
  line L396 (11.2932, -0.6397) -> (11.4702, -0.6397)
  line L397 (11.4702, -0.6397) -> (11.4702, -0.7554)
  spline S441 degree 2 poles (11.4702, -0.7554) (11.5394, -0.6862) (11.6755, -0.6102) (11.7572, -0.6102) knots 0 0 0 1 2 2 2
  spline S442 degree 2 poles (11.7572, -0.6102) (11.8502, -0.6102) (11.9943, -0.6953) (12.0318, -0.7918) knots 0 0 0 1 2 2 2
  spline S443 degree 2 poles (12.0318, -0.7918) (12.1123, -0.7021) (12.2643, -0.6102) (12.3528, -0.6102) knots 0 0 0 1 2 2 2
  spline S444 degree 2 poles (12.3528, -0.6102) (12.4209, -0.6102) (12.5321, -0.6522) (12.5729, -0.6999) knots 0 0 0 1 2 2 2
  spline S445 degree 2 poles (12.5729, -0.6999) (12.6149, -0.7475) (12.6614, -0.8905) (12.6614, -0.9982) knots 0 0 0 1 2 2 2
  line L398 (12.6614, -0.9982) -> (12.6614, -1.6903)
  line L399 (12.6614, -1.6903) -> (12.4844, -1.6903)
  line L400 (-12.4217, -2.761) -> (-13.0729, -2.761)
  line L401 (-13.0729, -2.761) -> (-13.0729, -3.1558)
  line L402 (-13.0729, -3.1558) -> (-12.449, -3.1558)
  line L403 (-12.449, -3.1558) -> (-12.449, -3.3215)
  line L404 (-12.449, -3.3215) -> (-13.0729, -3.3215)
  line L405 (-13.0729, -3.3215) -> (-13.0729, -3.9954)
  line L406 (-13.0729, -3.9954) -> (-13.259, -3.9954)
  line L407 (-13.259, -3.9954) -> (-13.259, -2.5954)
  line L408 (-13.259, -2.5954) -> (-12.4217, -2.5954)
  line L409 (-12.4217, -2.5954) -> (-12.4217, -2.761)
  line L410 (-12.0882, -3.9954) -> (-12.2652, -3.9954)
  line L411 (-12.2652, -3.9954) -> (-12.2652, -2.9448)
  line L412 (-12.2652, -2.9448) -> (-12.0882, -2.9448)
  line L413 (-12.0882, -2.9448) -> (-12.0882, -3.9954)
  line L414 (-12.0757, -2.7701) -> (-12.2765, -2.7701)
  line L415 (-12.2765, -2.7701) -> (-12.2765, -2.5863)
  line L416 (-12.2765, -2.5863) -> (-12.0757, -2.5863)
  line L417 (-12.0757, -2.5863) -> (-12.0757, -2.7701)
  spline S446 degree 2 poles (-10.948, -3.4531) (-10.948, -3.7106) (-11.1976, -4.0249) (-11.3859, -4.0249) knots 0 0 0 1 2 2 2
  spline S447 degree 2 poles (-11.3859, -4.0249) (-11.471, -4.0249) (-11.5924, -3.9829) (-11.6514, -3.9466) knots 0 0 0 1 2 2 2
  line L418 (-11.6514, -3.9466) -> (-11.6627, -3.9954)
  line L419 (-11.6627, -3.9954) -> (-11.8284, -3.9954)
  line L420 (-11.8284, -3.9954) -> (-11.8284, -2.533)
  line L421 (-11.8284, -2.533) -> (-11.6514, -2.533)
  line L422 (-11.6514, -2.533) -> (-11.6514, -3.0548)
  spline S448 degree 2 poles (-11.6514, -3.0548) (-11.5845, -2.9947) (-11.429, -2.9153) (-11.3303, -2.9153) knots 0 0 0 1 2 2 2
  spline S449 degree 2 poles (-11.3303, -2.9153) (-11.1522, -2.9153) (-10.948, -3.2001) (-10.948, -3.4531) knots 0 0 0 1 2 2 2
  spline S450 degree 2 poles (-11.1306, -3.4667) (-11.1306, -3.2783) (-11.2452, -3.0832) (-11.3723, -3.0832) knots 0 0 0 1 2 2 2
  spline S451 degree 2 poles (-11.3723, -3.0832) (-11.4438, -3.0832) (-11.5913, -3.1513) (-11.6514, -3.2035) knots 0 0 0 1 2 2 2
  line L423 (-11.6514, -3.2035) -> (-11.6514, -3.8059)
  spline S452 degree 2 poles (-11.6514, -3.8059) (-11.5845, -3.8388) (-11.4812, -3.866) (-11.4199, -3.866) knots 0 0 0 1 2 2 2
  spline S453 degree 2 poles (-11.4199, -3.866) (-11.2849, -3.866) (-11.1306, -3.6743) (-11.1306, -3.4667) knots 0 0 0 1 2 2 2
  spline S454 degree 2 poles (-10.3081, -4.0192) (-10.56, -4.0192) (-10.8368, -3.7367) (-10.8368, -3.4757) knots 0 0 0 1 2 2 2
  spline S455 degree 2 poles (-10.8368, -3.4757) (-10.8368, -3.2193) (-10.5679, -2.9153) (-10.3512, -2.9153) knots 0 0 0 1 2 2 2
  spline S456 degree 2 poles (-10.3512, -2.9153) (-10.2537, -2.9153) (-10.1028, -2.972) (-10.0472, -3.0321) knots 0 0 0 1 2 2 2
  spline S457 degree 2 poles (-10.0472, -3.0321) (-9.9905, -3.0923) (-9.9303, -3.2659) (-9.9303, -3.3918) knots 0 0 0 1 2 2 2
  line L424 (-9.9303, -3.3918) -> (-9.9303, -3.4882)
  line L425 (-9.9303, -3.4882) -> (-10.6576, -3.4882)
  spline S458 degree 2 poles (-10.6576, -3.4882) (-10.6576, -3.6709) (-10.4738, -3.8649) (-10.3104, -3.8649) knots 0 0 0 1 2 2 2
  spline S459 degree 2 poles (-10.3104, -3.8649) (-10.2525, -3.8649) (-10.1402, -3.8388) (-10.0948, -3.8184) knots 0 0 0 1 2 2 2
  spline S460 degree 2 poles (-10.0948, -3.8184) (-10.0472, -3.7957) (-9.9814, -3.756) (-9.9598, -3.7378) knots 0 0 0 1 2 2 2
  line L426 (-9.9598, -3.7378) -> (-9.9496, -3.7378)
  line L427 (-9.9496, -3.7378) -> (-9.9496, -3.9307)
  spline S461 degree 2 poles (-9.9496, -3.9307) (-9.9802, -3.9432) (-10.0733, -3.9795) (-10.1096, -3.9897) knots 0 0 0 1 2 2 2
  spline S462 degree 2 poles (-10.1096, -3.9897) (-10.1606, -4.0044) (-10.2446, -4.0192) (-10.3081, -4.0192) knots 0 0 0 1 2 2 2
  spline S463 degree 2 poles (-10.1028, -3.3532) (-10.105, -3.2817) (-10.1345, -3.1774) (-10.1629, -3.1422) knots 0 0 0 1 2 2 2
  spline S464 degree 2 poles (-10.1629, -3.1422) (-10.1935, -3.1025) (-10.29, -3.0605) (-10.3614, -3.0605) knots 0 0 0 1 2 2 2
  spline S465 degree 2 poles (-10.3614, -3.0605) (-10.4318, -3.0605) (-10.5305, -3.1025) (-10.5713, -3.1433) knots 0 0 0 1 2 2 2
  spline S466 degree 2 poles (-10.5713, -3.1433) (-10.611, -3.1853) (-10.6519, -3.2863) (-10.6576, -3.3532) knots 0 0 0 1 2 2 2
  line L428 (-10.6576, -3.3532) -> (-10.1028, -3.3532)
  line L429 (-9.194, -3.1343) -> (-9.2031, -3.1343)
  spline S467 degree 2 poles (-9.2031, -3.1343) (-9.2235, -3.1286) (-9.2678, -3.1263) (-9.2984, -3.1263) knots 0 0 0 1 2 2 2
  spline S468 degree 2 poles (-9.2984, -3.1263) (-9.3699, -3.1263) (-9.5105, -3.1887) (-9.5741, -3.25) knots 0 0 0 1 2 2 2
  line L430 (-9.5741, -3.25) -> (-9.5741, -3.9954)
  line L431 (-9.5741, -3.9954) -> (-9.7511, -3.9954)
  line L432 (-9.7511, -3.9954) -> (-9.7511, -2.9448)
  line L433 (-9.7511, -2.9448) -> (-9.5741, -2.9448)
  line L434 (-9.5741, -2.9448) -> (-9.5741, -3.1014)
  spline S469 degree 2 poles (-9.5741, -3.1014) (-9.4776, -3.0151) (-9.3336, -2.9448) (-9.2655, -2.9448) knots 0 0 0 1 2 2 2
  spline S470 degree 2 poles (-9.2655, -2.9448) (-9.2383, -2.9448) (-9.211, -2.9471) (-9.194, -2.9505) knots 0 0 0 1 2 2 2
  line L435 (-9.194, -2.9505) -> (-9.194, -3.1343)
  spline S471 degree 2 poles (-7.4514, -2.7553) (-7.372, -2.8484) (-7.2835, -3.1206) (-7.2835, -3.2954) knots 0 0 0 1 2 2 2
  spline S472 degree 2 poles (-7.2835, -3.2954) (-7.2835, -3.4655) (-7.3697, -3.7412) (-7.4514, -3.8343) knots 0 0 0 1 2 2 2
  spline S473 degree 2 poles (-7.4514, -3.8343) (-7.5376, -3.9318) (-7.7657, -4.0249) (-7.9029, -4.0249) knots 0 0 0 1 2 2 2
  spline S474 degree 2 poles (-7.9029, -4.0249) (-8.0447, -4.0249) (-8.2717, -3.9284) (-8.3545, -3.8343) knots 0 0 0 1 2 2 2
  spline S475 degree 2 poles (-8.3545, -3.8343) (-8.435, -3.7412) (-8.5212, -3.4678) (-8.5212, -3.2954) knots 0 0 0 1 2 2 2
  spline S476 degree 2 poles (-8.5212, -3.2954) (-8.5212, -3.1195) (-8.4339, -2.8518) (-8.3533, -2.7553) knots 0 0 0 1 2 2 2
  spline S477 degree 2 poles (-8.3533, -2.7553) (-8.2717, -2.6623) (-8.0436, -2.5659) (-7.9029, -2.5659) knots 0 0 0 1 2 2 2
  spline S478 degree 2 poles (-7.9029, -2.5659) (-7.76, -2.5659) (-7.5308, -2.6657) (-7.4514, -2.7553) knots 0 0 0 1 2 2 2
  spline S479 degree 2 poles (-7.4775, -3.2954) (-7.4775, -3.1569) (-7.5376, -2.9425) (-7.5921, -2.8722) knots 0 0 0 1 2 2 2
  spline S480 degree 2 poles (-7.5921, -2.8722) (-7.6477, -2.7996) (-7.8042, -2.727) (-7.9018, -2.727) knots 0 0 0 1 2 2 2
  spline S481 degree 2 poles (-7.9018, -2.727) (-8.0028, -2.727) (-8.1548, -2.7973) (-8.2127, -2.8722) knots 0 0 0 1 2 2 2
  spline S482 degree 2 poles (-8.2127, -2.8722) (-8.2682, -2.9437) (-8.3272, -3.1592) (-8.3272, -3.2954) knots 0 0 0 1 2 2 2
  spline S483 degree 2 poles (-8.3272, -3.2954) (-8.3272, -3.571) (-8.0958, -3.8638) (-7.9018, -3.8638) knots 0 0 0 1 2 2 2
  spline S484 degree 2 poles (-7.9018, -3.8638) (-7.7078, -3.8638) (-7.4775, -3.571) (-7.4775, -3.2954) knots 0 0 0 1 2 2 2
  line L436 (-6.276, -3.9954) -> (-6.453, -3.9954)
  line L437 (-6.453, -3.9954) -> (-6.453, -3.8796)
  spline S485 degree 2 poles (-6.453, -3.8796) (-6.5347, -3.9511) (-6.6811, -4.0249) (-6.7718, -4.0249) knots 0 0 0 1 2 2 2
  spline S486 degree 2 poles (-6.7718, -4.0249) (-6.8399, -4.0249) (-6.9613, -3.9795) (-7.0055, -3.9307) knots 0 0 0 1 2 2 2
  spline S487 degree 2 poles (-7.0055, -3.9307) (-7.0509, -3.8819) (-7.1008, -3.7333) (-7.1008, -3.6266) knots 0 0 0 1 2 2 2
  line L438 (-7.1008, -3.6266) -> (-7.1008, -2.9448)
  line L439 (-7.1008, -2.9448) -> (-6.9238, -2.9448)
  line L440 (-6.9238, -2.9448) -> (-6.9238, -3.5438)
  spline S488 degree 2 poles (-6.9238, -3.5438) (-6.9238, -3.6278) (-6.9114, -3.7378) (-6.8898, -3.7787) knots 0 0 0 1 2 2 2
  spline S489 degree 2 poles (-6.8898, -3.7787) (-6.8682, -3.8195) (-6.7945, -3.8569) (-6.7253, -3.8569) knots 0 0 0 1 2 2 2
  spline S490 degree 2 poles (-6.7253, -3.8569) (-6.6606, -3.8569) (-6.5143, -3.7832) (-6.453, -3.7299) knots 0 0 0 1 2 2 2
  line L441 (-6.453, -3.7299) -> (-6.453, -2.9448)
  line L442 (-6.453, -2.9448) -> (-6.276, -2.9448)
  line L443 (-6.276, -2.9448) -> (-6.276, -3.9954)
  spline S491 degree 2 poles (-5.702, -4.0158) (-5.846, -4.0158) (-6.0083, -3.8513) (-6.0083, -3.6732) knots 0 0 0 1 2 2 2
  line L444 (-6.0083, -3.6732) -> (-6.0083, -3.0911)
  line L445 (-6.0083, -3.0911) -> (-6.1274, -3.0911)
  line L446 (-6.1274, -3.0911) -> (-6.1274, -2.9448)
  line L447 (-6.1274, -2.9448) -> (-6.0083, -2.9448)
  line L448 (-6.0083, -2.9448) -> (-6.0083, -2.643)
  line L449 (-6.0083, -2.643) -> (-5.8313, -2.643)
  line L450 (-5.8313, -2.643) -> (-5.8313, -2.9448)
  line L451 (-5.8313, -2.9448) -> (-5.5057, -2.9448)
  line L452 (-5.5057, -2.9448) -> (-5.5057, -3.0911)
  line L453 (-5.5057, -3.0911) -> (-5.8313, -3.0911)
  line L454 (-5.8313, -3.0911) -> (-5.8313, -3.5915)
  spline S492 degree 2 poles (-5.8313, -3.5915) (-5.8313, -3.6709) (-5.8256, -3.7582) (-5.8063, -3.7957) knots 0 0 0 1 2 2 2
  spline S493 degree 2 poles (-5.8063, -3.7957) (-5.7905, -3.8286) (-5.719, -3.8615) (-5.6577, -3.8615) knots 0 0 0 1 2 2 2
  spline S494 degree 2 poles (-5.6577, -3.8615) (-5.6146, -3.8615) (-5.534, -3.8354) (-5.5159, -3.8274) knots 0 0 0 1 2 2 2
  line L455 (-5.5159, -3.8274) -> (-5.5057, -3.8274)
  line L456 (-5.5057, -3.8274) -> (-5.5057, -3.9863)
  spline S495 degree 2 poles (-5.5057, -3.9863) (-5.5556, -3.9999) (-5.6577, -4.0158) (-5.702, -4.0158) knots 0 0 0 1 2 2 2
  spline S496 degree 2 poles (-4.4948, -3.4417) (-4.4948, -3.7049) (-4.7456, -4.0158) (-4.9373, -4.0158) knots 0 0 0 1 2 2 2
  spline S497 degree 2 poles (-4.9373, -4.0158) (-5.0156, -4.0158) (-5.1358, -3.9795) (-5.1982, -3.942) knots 0 0 0 1 2 2 2
  line L457 (-5.1982, -3.942) -> (-5.1982, -4.3822)
  line L458 (-5.1982, -4.3822) -> (-5.3752, -4.3822)
  line L459 (-5.3752, -4.3822) -> (-5.3752, -2.9448)
  line L460 (-5.3752, -2.9448) -> (-5.1982, -2.9448)
  line L461 (-5.1982, -2.9448) -> (-5.1982, -3.0548)
  spline S498 degree 2 poles (-5.1982, -3.0548) (-5.1324, -2.9947) (-4.9713, -2.9153) (-4.8772, -2.9153) knots 0 0 0 1 2 2 2
  spline S499 degree 2 poles (-4.8772, -2.9153) (-4.6968, -2.9153) (-4.4948, -3.2012) (-4.4948, -3.4417) knots 0 0 0 1 2 2 2
  spline S500 degree 2 poles (-4.6775, -3.4621) (-4.6775, -3.2817) (-4.7921, -3.0832) (-4.9203, -3.0832) knots 0 0 0 1 2 2 2
  spline S501 degree 2 poles (-4.9203, -3.0832) (-4.9952, -3.0832) (-5.1358, -3.1501) (-5.1982, -3.2023) knots 0 0 0 1 2 2 2
  line L462 (-5.1982, -3.2023) -> (-5.1982, -3.7991)
  spline S502 degree 2 poles (-5.1982, -3.7991) (-5.129, -3.832) (-5.0303, -3.8569) (-4.9668, -3.8569) knots 0 0 0 1 2 2 2
  spline S503 degree 2 poles (-4.9668, -3.8569) (-4.8295, -3.8569) (-4.6775, -3.655) (-4.6775, -3.4621) knots 0 0 0 1 2 2 2
  line L463 (-3.4942, -3.9954) -> (-3.6712, -3.9954)
  line L464 (-3.6712, -3.9954) -> (-3.6712, -3.8796)
  spline S504 degree 2 poles (-3.6712, -3.8796) (-3.7529, -3.9511) (-3.8992, -4.0249) (-3.99, -4.0249) knots 0 0 0 1 2 2 2
  spline S505 degree 2 poles (-3.99, -4.0249) (-4.058, -4.0249) (-4.1794, -3.9795) (-4.2237, -3.9307) knots 0 0 0 1 2 2 2
  spline S506 degree 2 poles (-4.2237, -3.9307) (-4.2691, -3.8819) (-4.319, -3.7333) (-4.319, -3.6266) knots 0 0 0 1 2 2 2
  line L465 (-4.319, -3.6266) -> (-4.319, -2.9448)
  line L466 (-4.319, -2.9448) -> (-4.142, -2.9448)
  line L467 (-4.142, -2.9448) -> (-4.142, -3.5438)
  spline S507 degree 2 poles (-4.142, -3.5438) (-4.142, -3.6278) (-4.1295, -3.7378) (-4.108, -3.7787) knots 0 0 0 1 2 2 2
  spline S508 degree 2 poles (-4.108, -3.7787) (-4.0864, -3.8195) (-4.0127, -3.8569) (-3.9435, -3.8569) knots 0 0 0 1 2 2 2
  spline S509 degree 2 poles (-3.9435, -3.8569) (-3.8788, -3.8569) (-3.7324, -3.7832) (-3.6712, -3.7299) knots 0 0 0 1 2 2 2
  line L468 (-3.6712, -3.7299) -> (-3.6712, -2.9448)
  line L469 (-3.6712, -2.9448) -> (-3.4942, -2.9448)
  line L470 (-3.4942, -2.9448) -> (-3.4942, -3.9954)
  spline S510 degree 2 poles (-2.9201, -4.0158) (-3.0642, -4.0158) (-3.2264, -3.8513) (-3.2264, -3.6732) knots 0 0 0 1 2 2 2
  line L471 (-3.2264, -3.6732) -> (-3.2264, -3.0911)
  line L472 (-3.2264, -3.0911) -> (-3.3456, -3.0911)
  line L473 (-3.3456, -3.0911) -> (-3.3456, -2.9448)
  line L474 (-3.3456, -2.9448) -> (-3.2264, -2.9448)
  line L475 (-3.2264, -2.9448) -> (-3.2264, -2.643)
  line L476 (-3.2264, -2.643) -> (-3.0494, -2.643)
  line L477 (-3.0494, -2.643) -> (-3.0494, -2.9448)
  line L478 (-3.0494, -2.9448) -> (-2.7238, -2.9448)
  line L479 (-2.7238, -2.9448) -> (-2.7238, -3.0911)
  line L480 (-2.7238, -3.0911) -> (-3.0494, -3.0911)
  line L481 (-3.0494, -3.0911) -> (-3.0494, -3.5915)
  spline S511 degree 2 poles (-3.0494, -3.5915) (-3.0494, -3.6709) (-3.0438, -3.7582) (-3.0245, -3.7957) knots 0 0 0 1 2 2 2
  spline S512 degree 2 poles (-3.0245, -3.7957) (-3.0086, -3.8286) (-2.9371, -3.8615) (-2.8759, -3.8615) knots 0 0 0 1 2 2 2
  spline S513 degree 2 poles (-2.8759, -3.8615) (-2.8328, -3.8615) (-2.7522, -3.8354) (-2.734, -3.8274) knots 0 0 0 1 2 2 2
  line L482 (-2.734, -3.8274) -> (-2.7238, -3.8274)
  line L483 (-2.7238, -3.8274) -> (-2.7238, -3.9863)
  spline S514 degree 2 poles (-2.7238, -3.9863) (-2.7738, -3.9999) (-2.8759, -4.0158) (-2.9201, -4.0158) knots 0 0 0 1 2 2 2
  spline S515 degree 2 poles (-1.0935, -3.0174) (-1.0935, -3.1082) (-1.1582, -3.2715) (-1.2161, -3.3283) knots 0 0 0 1 2 2 2
  spline S516 degree 2 poles (-1.2161, -3.3283) (-1.2887, -3.3997) (-1.4849, -3.4735) (-1.6347, -3.4735) knots 0 0 0 1 2 2 2
  line L484 (-1.6347, -3.4735) -> (-1.7924, -3.4735)
  line L485 (-1.7924, -3.4735) -> (-1.7924, -3.9954)
  line L486 (-1.7924, -3.9954) -> (-1.9785, -3.9954)
  line L487 (-1.9785, -3.9954) -> (-1.9785, -2.5954)
  line L488 (-1.9785, -2.5954) -> (-1.6268, -2.5954)
  spline S517 degree 2 poles (-1.6268, -2.5954) (-1.502, -2.5954) (-1.3272, -2.6362) (-1.2603, -2.6827) knots 0 0 0 1 2 2 2
  spline S518 degree 2 poles (-1.2603, -2.6827) (-1.182, -2.736) (-1.0935, -2.9005) (-1.0935, -3.0174) knots 0 0 0 1 2 2 2
  spline S519 degree 2 poles (-1.2875, -3.0231) (-1.2875, -2.9505) (-1.3375, -2.8438) (-1.3885, -2.8098) knots 0 0 0 1 2 2 2
  spline S520 degree 2 poles (-1.3885, -2.8098) (-1.4328, -2.7803) (-1.5507, -2.7565) (-1.6381, -2.7565) knots 0 0 0 1 2 2 2
  line L489 (-1.6381, -2.7565) -> (-1.7924, -2.7565)
  line L490 (-1.7924, -2.7565) -> (-1.7924, -3.3146)
  line L491 (-1.7924, -3.3146) -> (-1.6653, -3.3146)
  spline S521 degree 2 poles (-1.6653, -3.3146) (-1.5519, -3.3146) (-1.4123, -3.2783) (-1.367, -3.2307) knots 0 0 0 1 2 2 2
  spline S522 degree 2 poles (-1.367, -3.2307) (-1.325, -3.1887) (-1.2875, -3.09) (-1.2875, -3.0231) knots 0 0 0 1 2 2 2
  spline S523 degree 2 poles (-0.0668, -3.4701) (-0.0668, -3.7356) (-0.3221, -4.0249) (-0.5353, -4.0249) knots 0 0 0 1 2 2 2
  spline S524 degree 2 poles (-0.5353, -4.0249) (-0.7543, -4.0249) (-1.005, -3.7265) (-1.005, -3.4701) knots 0 0 0 1 2 2 2
  spline S525 degree 2 poles (-1.005, -3.4701) (-1.005, -3.2069) (-0.7464, -2.9153) (-0.5353, -2.9153) knots 0 0 0 1 2 2 2
  spline S526 degree 2 poles (-0.5353, -2.9153) (-0.3221, -2.9153) (-0.0668, -3.2057) (-0.0668, -3.4701) knots 0 0 0 1 2 2 2
  spline S527 degree 2 poles (-0.2494, -3.4701) (-0.2494, -3.2659) (-0.3981, -3.0673) (-0.5353, -3.0673) knots 0 0 0 1 2 2 2
  spline S528 degree 2 poles (-0.5353, -3.0673) (-0.6726, -3.0673) (-0.8224, -3.2659) (-0.8224, -3.4701) knots 0 0 0 1 2 2 2
  spline S529 degree 2 poles (-0.8224, -3.4701) (-0.8224, -3.6686) (-0.6726, -3.8728) (-0.5353, -3.8728) knots 0 0 0 1 2 2 2
  spline S530 degree 2 poles (-0.5353, -3.8728) (-0.3992, -3.8728) (-0.2494, -3.672) (-0.2494, -3.4701) knots 0 0 0 1 2 2 2
  line L492 (1.3877, -2.9448) -> (1.1211, -3.9954)
  line L493 (1.1211, -3.9954) -> (0.9577, -3.9954)
  line L494 (0.9577, -3.9954) -> (0.7013, -3.1853)
  line L495 (0.7013, -3.1853) -> (0.446, -3.9954)
  line L496 (0.446, -3.9954) -> (0.2838, -3.9954)
  line L497 (0.2838, -3.9954) -> (0.0149, -2.9448)
  line L498 (0.0149, -2.9448) -> (0.1987, -2.9448)
  line L499 (0.1987, -2.9448) -> (0.3848, -3.7582)
  line L500 (0.3848, -3.7582) -> (0.6332, -2.9448)
  line L501 (0.6332, -2.9448) -> (0.7796, -2.9448)
  line L502 (0.7796, -2.9448) -> (1.0348, -3.7582)
  line L503 (1.0348, -3.7582) -> (1.2095, -2.9448)
  line L504 (1.2095, -2.9448) -> (1.3877, -2.9448)
  spline S531 degree 2 poles (1.9992, -4.0192) (1.7473, -4.0192) (1.4705, -3.7367) (1.4705, -3.4757) knots 0 0 0 1 2 2 2
  spline S532 degree 2 poles (1.4705, -3.4757) (1.4705, -3.2193) (1.7394, -2.9153) (1.9561, -2.9153) knots 0 0 0 1 2 2 2
  spline S533 degree 2 poles (1.9561, -2.9153) (2.0536, -2.9153) (2.2045, -2.972) (2.2601, -3.0321) knots 0 0 0 1 2 2 2
  spline S534 degree 2 poles (2.2601, -3.0321) (2.3168, -3.0923) (2.377, -3.2659) (2.377, -3.3918) knots 0 0 0 1 2 2 2
  line L505 (2.377, -3.3918) -> (2.377, -3.4882)
  line L506 (2.377, -3.4882) -> (1.6497, -3.4882)
  spline S535 degree 2 poles (1.6497, -3.4882) (1.6497, -3.6709) (1.8335, -3.8649) (1.9969, -3.8649) knots 0 0 0 1 2 2 2
  spline S536 degree 2 poles (1.9969, -3.8649) (2.0548, -3.8649) (2.1671, -3.8388) (2.2125, -3.8184) knots 0 0 0 1 2 2 2
  spline S537 degree 2 poles (2.2125, -3.8184) (2.2601, -3.7957) (2.3259, -3.756) (2.3475, -3.7378) knots 0 0 0 1 2 2 2
  line L507 (2.3475, -3.7378) -> (2.3577, -3.7378)
  line L508 (2.3577, -3.7378) -> (2.3577, -3.9307)
  spline S538 degree 2 poles (2.3577, -3.9307) (2.3271, -3.9432) (2.234, -3.9795) (2.1977, -3.9897) knots 0 0 0 1 2 2 2
  spline S539 degree 2 poles (2.1977, -3.9897) (2.1467, -4.0044) (2.0627, -4.0192) (1.9992, -4.0192) knots 0 0 0 1 2 2 2
  spline S540 degree 2 poles (2.2045, -3.3532) (2.2023, -3.2817) (2.1728, -3.1774) (2.1444, -3.1422) knots 0 0 0 1 2 2 2
  spline S541 degree 2 poles (2.1444, -3.1422) (2.1138, -3.1025) (2.0173, -3.0605) (1.9459, -3.0605) knots 0 0 0 1 2 2 2
  spline S542 degree 2 poles (1.9459, -3.0605) (1.8755, -3.0605) (1.7768, -3.1025) (1.736, -3.1433) knots 0 0 0 1 2 2 2
  spline S543 degree 2 poles (1.736, -3.1433) (1.6963, -3.1853) (1.6554, -3.2863) (1.6497, -3.3532) knots 0 0 0 1 2 2 2
  line L509 (1.6497, -3.3532) -> (2.2045, -3.3532)
  line L510 (3.1133, -3.1343) -> (3.1042, -3.1343)
  spline S544 degree 2 poles (3.1042, -3.1343) (3.0838, -3.1286) (3.0395, -3.1263) (3.0089, -3.1263) knots 0 0 0 1 2 2 2
  spline S545 degree 2 poles (3.0089, -3.1263) (2.9374, -3.1263) (2.7967, -3.1887) (2.7332, -3.25) knots 0 0 0 1 2 2 2
  line L511 (2.7332, -3.25) -> (2.7332, -3.9954)
  line L512 (2.7332, -3.9954) -> (2.5562, -3.9954)
  line L513 (2.5562, -3.9954) -> (2.5562, -2.9448)
  line L514 (2.5562, -2.9448) -> (2.7332, -2.9448)
  line L515 (2.7332, -2.9448) -> (2.7332, -3.1014)
  spline S546 degree 2 poles (2.7332, -3.1014) (2.8296, -3.0151) (2.9737, -2.9448) (3.0418, -2.9448) knots 0 0 0 1 2 2 2
  spline S547 degree 2 poles (3.0418, -2.9448) (3.069, -2.9448) (3.0963, -2.9471) (3.1133, -2.9505) knots 0 0 0 1 2 2 2
  line L516 (3.1133, -2.9505) -> (3.1133, -3.1343)
  line L517 (4.1763, -3.2125) -> (3.9517, -3.2125)
  line L518 (3.9517, -3.2125) -> (3.9517, -2.9448)
  line L519 (3.9517, -2.9448) -> (4.1763, -2.9448)
  line L520 (4.1763, -2.9448) -> (4.1763, -3.2125)
  line L521 (4.1763, -3.9954) -> (3.9517, -3.9954)
  line L522 (3.9517, -3.9954) -> (3.9517, -3.7276)
  line L523 (3.9517, -3.7276) -> (4.1763, -3.7276)
  line L524 (4.1763, -3.7276) -> (4.1763, -3.9954)
  spline S548 degree 2 poles (5.5309, -4.0271) (5.4266, -4.0271) (5.2553, -3.9647) (5.1951, -3.9069) knots 0 0 0 1 2 2 2
  spline S549 degree 2 poles (5.1951, -3.9069) (5.1361, -3.8501) (5.0749, -3.6958) (5.0749, -3.6085) knots 0 0 0 1 2 2 2
  spline S550 degree 2 poles (5.0749, -3.6085) (5.0749, -3.495) (5.1963, -3.3044) (5.312, -3.2477) knots 0 0 0 1 2 2 2
  line L525 (5.312, -3.2477) -> (5.312, -3.242)
  spline S551 degree 2 poles (5.312, -3.242) (5.2087, -3.1819) (5.1089, -3.039) (5.1089, -2.9323) knots 0 0 0 1 2 2 2
  spline S552 degree 2 poles (5.1089, -2.9323) (5.1089, -2.7746) (5.3471, -2.5636) (5.5309, -2.5636) knots 0 0 0 1 2 2 2
  spline S553 degree 2 poles (5.5309, -2.5636) (5.7215, -2.5636) (5.9518, -2.7633) (5.9518, -2.9198) knots 0 0 0 1 2 2 2
  spline S554 degree 2 poles (5.9518, -2.9198) (5.9518, -3.014) (5.8418, -3.1978) (5.7386, -3.25) knots 0 0 0 1 2 2 2
  line L526 (5.7386, -3.25) -> (5.7386, -3.2556)
  spline S555 degree 2 poles (5.7386, -3.2556) (5.8611, -3.3124) (5.987, -3.4757) (5.987, -3.6051) knots 0 0 0 1 2 2 2
  spline S556 degree 2 poles (5.987, -3.6051) (5.987, -3.7843) (5.7261, -4.0271) (5.5309, -4.0271) knots 0 0 0 1 2 2 2
  spline S557 degree 2 poles (5.7942, -3.6232) (5.7942, -3.537) (5.7261, -3.4349) (5.6296, -3.3827) knots 0 0 0 1 2 2 2
  spline S558 degree 2 poles (5.6296, -3.3827) (5.5979, -3.3646) (5.4912, -3.3226) (5.4243, -3.2954) knots 0 0 0 1 2 2 2
  spline S559 degree 2 poles (5.4243, -3.2954) (5.3471, -3.3464) (5.2643, -3.4984) (5.2643, -3.5949) knots 0 0 0 1 2 2 2
  spline S560 degree 2 poles (5.2643, -3.5949) (5.2643, -3.7219) (5.4175, -3.8876) (5.5332, -3.8876) knots 0 0 0 1 2 2 2
  spline S561 degree 2 poles (5.5332, -3.8876) (5.6512, -3.8876) (5.7942, -3.7458) (5.7942, -3.6232) knots 0 0 0 1 2 2 2
  spline S562 degree 2 poles (5.7681, -2.9221) (5.7681, -2.8279) (5.6421, -2.702) (5.5298, -2.702) knots 0 0 0 1 2 2 2
  spline S563 degree 2 poles (5.5298, -2.702) (5.4277, -2.702) (5.2972, -2.8143) (5.2972, -2.9108) knots 0 0 0 1 2 2 2
  spline S564 degree 2 poles (5.2972, -2.9108) (5.2972, -2.98) (5.3642, -3.0764) (5.4311, -3.115) knots 0 0 0 1 2 2 2
  spline S565 degree 2 poles (5.4311, -3.115) (5.4595, -3.1309) (5.5797, -3.1864) (5.6285, -3.2023) knots 0 0 0 1 2 2 2
  spline S566 degree 2 poles (5.6285, -3.2023) (5.7102, -3.1399) (5.7681, -3.0072) (5.7681, -2.9221) knots 0 0 0 1 2 2 2
  line L527 (6.459, -3.9954) -> (6.2343, -3.9954)
  line L528 (6.2343, -3.9954) -> (6.2343, -3.7276)
  line L529 (6.2343, -3.7276) -> (6.459, -3.7276)
  line L530 (6.459, -3.7276) -> (6.459, -3.9954)
  spline S567 degree 2 poles (7.6128, -3.2954) (7.6128, -3.672) (7.3938, -4.0249) (7.1658, -4.0249) knots 0 0 0 1 2 2 2
  spline S568 degree 2 poles (7.1658, -4.0249) (6.9343, -4.0249) (6.7177, -3.6652) (6.7177, -3.2965) knots 0 0 0 1 2 2 2
  spline S569 degree 2 poles (6.7177, -3.2965) (6.7177, -2.9176) (6.9366, -2.567) (7.1658, -2.567) knots 0 0 0 1 2 2 2
  spline S570 degree 2 poles (7.1658, -2.567) (7.3961, -2.567) (7.6128, -2.93) (7.6128, -3.2954) knots 0 0 0 1 2 2 2
  spline S571 degree 2 poles (7.3723, -3.7219) (7.3995, -3.6527) (7.4222, -3.4394) (7.4222, -3.2954) knots 0 0 0 1 2 2 2
  spline S572 degree 2 poles (7.4222, -3.2954) (7.4222, -3.1513) (7.3995, -2.9391) (7.3711, -2.8676) knots 0 0 0 1 2 2 2
  spline S573 degree 2 poles (7.3711, -2.8676) (7.3428, -2.7962) (7.2441, -2.7224) (7.1658, -2.7224) knots 0 0 0 1 2 2 2
  spline S574 degree 2 poles (7.1658, -2.7224) (7.0875, -2.7224) (6.9865, -2.7962) (6.957, -2.8699) knots 0 0 0 1 2 2 2
  spline S575 degree 2 poles (6.957, -2.8699) (6.9287, -2.9414) (6.9083, -3.1592) (6.9083, -3.2965) knots 0 0 0 1 2 2 2
  spline S576 degree 2 poles (6.9083, -3.2965) (6.9083, -3.444) (6.9264, -3.6414) (6.9559, -3.7185) knots 0 0 0 1 2 2 2
  spline S577 degree 2 poles (6.9559, -3.7185) (6.9831, -3.7911) (7.0841, -3.8694) (7.1658, -3.8694) knots 0 0 0 1 2 2 2
  spline S578 degree 2 poles (7.1658, -3.8694) (7.2429, -3.8694) (7.3439, -3.7957) (7.3723, -3.7219) knots 0 0 0 1 2 2 2
  line L531 (9.6107, -3.9954) -> (9.6107, -3.3873)
  spline S579 degree 2 poles (9.6107, -3.3873) (9.6107, -3.3146) (9.5993, -3.191) (9.5812, -3.1569) knots 0 0 0 1 2 2 2
  spline S580 degree 2 poles (9.5812, -3.1569) (9.563, -3.1195) (9.4938, -3.0832) (9.4337, -3.0832) knots 0 0 0 1 2 2 2